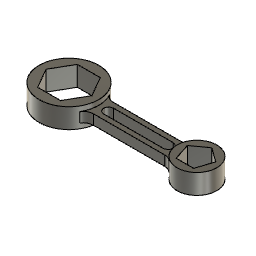
Exercise_2 (Autodesk Fusion 360 design; units mm, degrees)
Autodesk Fusion 360 part; units mm, degrees
sketch "Sketch1" plane through (0, 0, 0) normal (0, 0, 1) x (1, 0, 0)
  circle A0 centre (0, 0) radius 30
  circle A1 centre (129, 0) radius 20
  dimension "d1" = 60
  dimension "d2" = 40
  dimension "d3" = 129
  constraint coincident A0.centre origin
  constraint horizontal A0.centre A1.centre
  measures "d1" diameter of A0
  measures "d2" diameter of A1
  measures "d3" distance of A0.centre A1.centre
extrude "Extrude1" add sketch "Sketch1" along normal blind 10 and the other way blind 10 makes body 1 at (123.4917, 3.7555, 10) makes body 2 at (1.8926, -11.2064, 10)
sketch "Sketch2" plane through (0, 0, 0) normal (0, 0, 1) x (1, 0, 0)
  line L0 (0, 10) -> (111.6795, 10)
  line L1 (111.6795, 10) -> (111.6795, -10)
  line L2 (111.6795, -10) -> (0, -10)
  line L3 (0, -10) -> (0, 10)
  circle A0 centre (129, 0) radius 20
  dimension "d8" = 20
  constraint horizontal L0
  constraint vertical L1
  constraint horizontal L2
  constraint vertical L3
  constraint midpoint origin L3
  constraint coincident L0.end A0
  measures "d8" distance of L0.end L1.end
extrude "Extrude2" add sketch "Sketch2" along normal blind 5 and the other way blind 5 contours L0 L2 L3 A0 bodies 2 1
fillet "Fillet1" radius 10 4 edges at (28.2843, 10, 0) (28.2843, -10, 0) (111.6795, -10, 0) (111.6795, 10, 0) on bodies 2
sketch "Sketch3" plane through (0, 0, 10) normal (0, 0, 1) x (-1, 0, 0)
  circle A0 centre (-129, 0) radius 20
  line L0 (-11.547, 20) -> (-23.094, 0)
  line L1 (-23.094, 0) -> (-11.547, -20)
  line L2 (-11.547, -20) -> (11.547, -20)
  line L3 (11.547, -20) -> (23.094, 0)
  line L4 (23.094, 0) -> (11.547, 20)
  line L5 (11.547, 20) -> (-11.547, 20)
  line L6 (-137.8168, 12.1353) -> (-143.2658, -4.6353)
  line L7 (-143.2658, -4.6353) -> (-129, -15)
  line L8 (-129, -15) -> (-114.7342, -4.6353)
  line L9 (-114.7342, -4.6353) -> (-120.1832, 12.1353)
  line L10 (-120.1832, 12.1353) -> (-137.8168, 12.1353)
  line L11 (-38, 0) -> (-98, 0) construction
  point P0 (-129, 0)
  dimension "d14" = 20
  dimension "d15" = 15
  constraint vertical P0 A0.centre
  constraint coincident P0 A0.centre
  constraint horizontal L11
  constraint horizontal P0 L11.end
  constraint vertical L7.end P0
  constraint horizontal origin L0.end
  measures "d14" distance of origin L2
  measures "d15" distance of L7.end P0
extrude "Extrude3" cut sketch "Sketch3" against normal blind 20 contours L0 L1 L2 L3 L4 L5 | L6 L7 L8 L9 L10 bodies 2
sketch "Sketch4" plane through (0, 0, 5) normal (0, 0, 1) x (-1, 0, 0)
  arc A0 (-25.9808, 15) -> (-25.9808, -15) centre (0, 0) ccw
  arc A1 (-34.641, 10) -> (-25.9808, 15) centre (-34.641, 20) ccw
  line L0 (-34.641, 10) -> (-106.6393, 10)
  arc A2 (-114.0929, 13.3333) -> (-106.6393, 10) centre (-106.6393, 20) ccw
  arc A3 (-114.0929, -13.3333) -> (-114.0929, 13.3333) centre (-129, 0) ccw
  arc A4 (-106.6393, -10) -> (-114.0929, -13.3333) centre (-106.6393, -20) ccw
  line L1 (-106.6393, -10) -> (-34.641, -10)
  arc A5 (-25.9808, -15) -> (-34.641, -10) centre (-34.641, -20) ccw
  line L2 (-40, 5) -> (-100, 5)
  arc A6 (-100, 5) -> (-100, -5) centre (-100, 0) ccw
  line L3 (-100, -5) -> (-40, -5)
  arc A7 (-40, -5) -> (-40, 5) centre (-40, 0) ccw
  line L4 (-40, 0) -> (-100, 0) construction
  dimension "d21" = 60
  dimension "d22" = 10
  dimension "d23" = 40
  constraint tangent L2 A6
  constraint tangent A6 L3
  constraint parallel L2 L3
  constraint tangent L3 A7
  constraint tangent L2 A7
  constraint horizontal L4
  constraint horizontal A3.centre A6.centre
  measures "d21" distance of A7.centre A6.centre
  measures "d22" distance of L2 L3
  measures "d23" distance of A0.centre A7.centre
extrude "Extrude4" cut sketch "Sketch4" against normal blind 10 contours L2 A6 L3 A7 bodies 2
